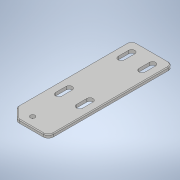
# Autodesk Inventor part: Rear
Saved by Autodesk Inventor 2021 (Build 250183000, 183)
## iProperties
Created: 2021-02-16
Part Number: Rear
Material: Generic
Document SubType Name: Modeling
Designer: Viktor
Density: 1 g/cm^3
Appearance: Default
Author: Viktor
Autodesk Inventor part; units mm, degrees
ref_plane "YZ Plane" through (0, 0, 0) normal (1, 0, 0) x (0, 1, 0)
ref_plane "XZ Plane" through (0, 0, 0) normal (0, 1, 0) x (-1, 0, 0)
ref_plane "XY Plane" through (0, 0, 0) normal (0, 0, 1) x (1, 0, 0)
sketch "Sketch1" plane through (0, 0, 0) normal (0, 1, 0) x (-1, 0, 0)
  line L0 (-20, 60) -> (20, 60)
  line L1 (20, 60) -> (20, -60)
  line L2 (20, -60) -> (-20, -60)
  line L3 (-20, -60) -> (-20, 60)
  line L4 (-20, 60) -> (20, -60) construction
  line L5 (20, 60) -> (-20, -60) construction
  point P0 (0, 0)
  dimension "d0" = 120
  dimension "d1" = 40
  constraints: 12 end point, 2 midpoint, 2 parallel, 1 horizontal, 1 perpendicular
  measures "d0" distance of L0.end L1.end
  measures "d1" distance of L1.end L2.end
extrude "Extrusion1" add sketch "Sketch1" along normal blind 3
sketch "Sketch2" plane through (0, 3, 0) normal (0, 1, 0) x (1, 0, 0)
  line L0 (-10, -20) -> (-10, -10) construction
  line L1 (-7, -20) -> (-7, -10)
  line L2 (-13, -10) -> (-13, -20)
  arc A0 (-13, -20) -> (-7, -20) centre (-10, -20) ccw
  arc A1 (-7, -10) -> (-13, -10) centre (-10, -10) ccw
  line L3 (-32, 15) -> (32, 15) construction
  line L4 (20, 60) -> (-20, 60) projected
  line L5 (0, 84) -> (0, -84) projected
  line L6 (-10, 50) -> (-10, 40) construction
  line L7 (-7, 50) -> (-7, 40)
  line L8 (-13, 40) -> (-13, 50)
  arc A2 (-7, 50) -> (-13, 50) centre (-10, 50) ccw
  arc A3 (-13, 40) -> (-7, 40) centre (-10, 40) ccw
  line L9 (10, -20) -> (10, -10) construction
  line L10 (7, -20) -> (7, -10)
  line L11 (13, -10) -> (13, -20)
  arc A4 (7, -20) -> (13, -20) centre (10, -20) ccw
  arc A5 (13, -10) -> (7, -10) centre (10, -10) ccw
  line L12 (10, 50) -> (10, 40) construction
  line L13 (7, 50) -> (7, 40)
  line L14 (13, 40) -> (13, 50)
  arc A6 (13, 50) -> (7, 50) centre (10, 50) ccw
  arc A7 (7, 40) -> (13, 40) centre (10, 40) ccw
  point P0 (0, 0)
  point P1 (-10, -15)
  point P2 (-10, 45)
  point P3 (10, -15)
  point P4 (10, 45)
  dimension "d4" = 3
  dimension "d5" = 10
  dimension "d6" = 30
  dimension "d7" = 45
  dimension "d8" = 10
  constraints: 34 end point, 21 symmetric about line, 16 point on circle, 8 centre point, 4 tangent, 1 horizontal, 1 midpoint, 1 parallel, 1 vertical, 6 other
  measures "d4" radius of A1
  measures "d5" distance of L2.start L2.end
  measures "d6" distance from line of L3 point (-10, -15)
  measures "d7" distance between parallel lines of L4 L3
  measures "d8" distance from line of L5 point (-10, -15)
sketch "Sketch3" plane through (0, 3, 0) normal (0, 1, 0) x (1, 0, 0)
  circle A0 centre (-4, -51) radius 2.25
  line L0 (-20, -60) -> (20, -60) projected
  line L1 (20, -60) -> (20, 60) projected
  line L2 (-20, 60) -> (-20, -60) projected
  point P0 (0, 0)
  dimension "d9" = 4.5
  dimension "d10" = 9
  dimension "d16" = 16
  constraints: 1 centre point
  measures "d9" diameter of A0
  measures "d10" distance from line of L0 A0.centre
  measures "d16" distance from line of L2 A0.centre
extrude "Extrusion2" cut sketch "Sketch3" against normal blind 3
extrude "Extrusion3" cut sketch "Sketch2" against normal blind 3
chamfer "Chamfer1" distance 10 angle 45 1 edges at (-20, 1.5, 60)
fillet "Fillet1" radius 5 5 edges at (-10, 1.5, 60) (-20, 1.5, 50) (20, 1.5, 60) (20, 1.5, -60) (-20, 1.5, -60)
chamfer "Chamfer2" distance 0.75 angle 45 10 edges at (20, 3, 0) (18.5355, 3, -58.5355) (0, 3, -60) (-18.5355, 3, -58.5355) (-20, 3, -3.5355) (-19.6194, 3, 49.8423) (-15, 3, 55) (-9.8423, 3, 59.6194) (3.5355, 3, 60) (18.5355, 3, 58.5355)
body "Solid1"
